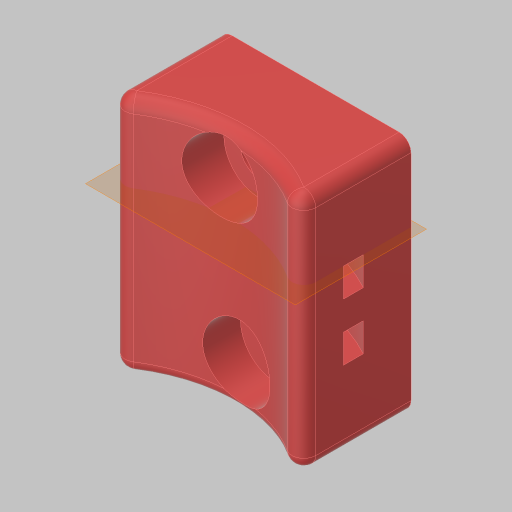
# Autodesk Inventor part: WL-009
Saved by Autodesk Inventor 2023.5 (Build 275446000, 446)
## iProperties
Created: 2025-03-02
Part Number: WL-009
Material: ABS Plastic
Document SubType Name: Modeling
Designer: slick
Density: 1.06 g/cm^3
Appearance: Smooth - Red
Author: slick
Autodesk Inventor part; units mm, degrees
ref_plane "YZ Plane" through (0, 0, 0) normal (1, 0, 0) x (0, 1, 0)
ref_plane "XZ Plane" through (0, 0, 0) normal (0, 1, 0) x (-1, 0, 0)
ref_plane "XY Plane" through (0, 0, 0) normal (0, 0, 1) x (1, 0, 0)
sketch "Sketch1" plane through (0, 0, 0) normal (0, 0, 1) x (1, 0, 0)
  line L0 (-12.7, -15.875) -> (12.7, -15.875)
  line L1 (12.7, -15.875) -> (12.7, 15.875)
  line L2 (12.7, 15.875) -> (-12.7, 15.875)
  line L3 (-12.7, 15.875) -> (-12.7, -15.875)
  line L4 (-12.7, -15.875) -> (12.7, 15.875) construction
  line L5 (12.7, -15.875) -> (-12.7, 15.875) construction
  line L6 (-1.1061, 10.0868) -> (1.1061, -10.0868) construction
  point P0 (0, 0)
  dimension "d0" = 31.75
  dimension "d1" = 25.4
  dimension "d2" = 2.2121
  dimension "d3" = 20.1737
  constraints: 14 end point, 3 midpoint, 2 parallel, 1 horizontal, 1 perpendicular
  measures "d0" distance of L2.end L0.start
  measures "d1" distance of L1.end L2.end
  measures "d2" horizontal distance of L6.start L6.end
  measures "d3" vertical distance of L6.end L6.start
extrude "Extrusion1" add sketch "Sketch1" along normal blind 19.05
sketch "Sketch2" plane through (-12.7, 15.875, 0) normal (0, 1, 0) x (1, 0, 0)
  line L0 (25.4, 0) -> (0, 0) projected
  line L1 (0, 0) -> (0, -19.05) projected
  line L2 (25.4, -19.05) -> (0, -19.05) projected
  line L3 (25.4, 0) -> (25.4, -19.05) projected
  line L4 (25.4, 0) -> (25.4, -19.05) construction
  line L5 (0, 0) -> (0, -19.05) construction
  arc A0 (25.4, -15.875) -> (0, -15.875) centre (12.7, -30.074) ccw
  point P0 (12.7, 0)
  point P1 (0, -15.875)
  dimension "d13" = 19.05
  dimension "d14" = 3.175
  constraints: 2 point on circle, 2 point on line, 1 centre point, 1 horizontal alignment
  measures "d13" radius of A0
  measures "d14" distance of L1.end A0.end
extrude "Extrusion2" cut sketch "Sketch2" against normal through all contours L3 L2 L1 A0
ref_plane "Work Plane1" through (0, 0, 11.176) normal (0, 0, -1) x (-1, 0, 0)
sketch "Sketch3" plane through (0, 0, 11.176) normal (0, 0, -1) x (-1, 0, 0)
  line L0 (12.7, 15.875) -> (12.7, -15.875) construction
  line L1 (12.7, -15.875) -> (-12.7, -15.875) construction
  line L2 (-12.7, 15.875) -> (12.7, 15.875) construction
  line L3 (-12.7, -15.875) -> (-12.7, 15.875) construction
  line L4 (12.7, -15.875) -> (12.7, 15.875) construction
  line L5 (-12.7, 15.875) -> (12.7, 15.875) construction
  line L6 (-12.7, 15.875) -> (-12.7, -15.875) construction
  line L7 (12.7, -15.875) -> (-12.7, -15.875) construction
  line L8 (12.7, -15.875) -> (-12.7, -15.875) construction
  line L9 (-12.7, -15.875) -> (-12.7, 15.875) construction
  line L10 (-12.7, 15.875) -> (12.7, 15.875) construction
  line L11 (12.7, 15.875) -> (12.7, -15.875) construction
  line L12 (12.7, -15.875) -> (-12.7, 15.875) construction
  line L13 (-12.7, -15.875) -> (12.7, 15.875) construction
  line L14 (1.1061, 10.0868) -> (-1.1061, -10.0868) construction
  point P0 (0, 0)
  point P1 (0, 0)
  constraints: 2 coincident
hole "Hole2" at (-1.1061, 10.0868, 11.176) at (1.1061, -10.0868, 11.176) direction (0, 0, -1) diameter 5.1054 end through all start extended yes counterbore diameter 9.525 counterbore depth 4.826 clearance for "Socket Head Cap Screw" size "#10" standard "Ansi Unified Screw Threads"
ref_plane "Work Plane2" through (-12.7, 5.715, 0) normal (0, 1, 0) x (1, 0, 0)
sketch "Sketch5" plane through (-12.7, 5.715, 0) normal (0, 1, 0) x (1, 0, 0)
  line L0 (25.4, 0) -> (25.4, -15.875) construction
  line L1 (0, 0) -> (0, -15.875) construction
  arc A0 (25.4, -8.9784) -> (0, -8.9784) centre (12.7, -30.074) ccw
  arc A1 (25.4, -15.875) -> (0, -15.875) centre (12.7, -30.074) ccw construction
  arc A2 (25.4, -6.35) -> (0, -6.35) centre (12.7, -30.074) ccw
  line L2 (0, -6.35) -> (0, -8.9784)
  line L3 (25.4, -6.35) -> (25.4, -8.9784)
  point P0 (12.7, 0)
  dimension "d29" = 2.286
  dimension "d30" = 6.35
  constraints: 4 end point, 4 point on circle, 4 point on line, 2 centre point, 1 concentric, 1 parallel, 1 vertical
  measures "d29" radial gap between concentric circles of A0 A2
  measures "d30" distance of L1.start L2.start
extrude "Extrusion3" cut sketch "Sketch5" against normal blind 3.81
mirror "Mirror1" about plane through (0, 0, 0) normal (0, 1, 0) of "Extrusion3"
fillet "Fillet1" radius 1.5875 8 edges at (-12.7, 0, 15.875) (12.7, 0, 15.875) (0, 15.875, 11.024) (0, -15.875, 11.024) (-12.7, 15.875, 7.9375) (12.7, 15.875, 7.9375) (12.7, -15.875, 7.9375) (-12.7, -15.875, 7.9375)
body "Solid1"
